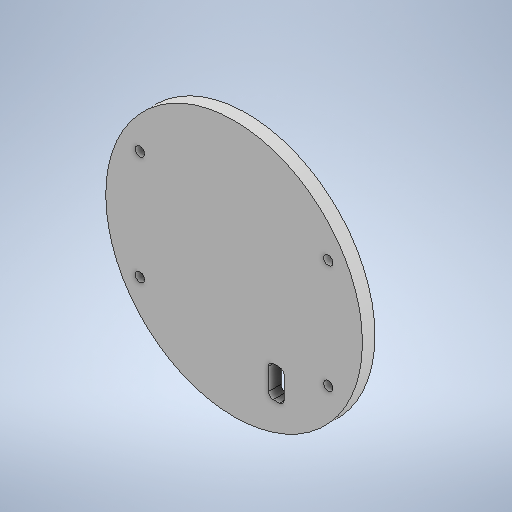
# Autodesk Inventor part: lower-plate
Saved by Autodesk Inventor 2025 (Build 290162000, 162)
## iProperties
Created: 2024-05-27
Part Number: lower-plate
Material: Generic
Document SubType Name: Modeling
Designer: hifzh
Density: 1 g/cm^3
Appearance: Default
Author: hifzh
## iProperties of the stored document lower-plate_3DPrint.ipt
Created: 2024-05-27
Part Number: lower-plate_3DPrint
Material: Generic
Document SubType Name: Modeling
Designer: hifzh
Density: 1 g/cm^3
Appearance: Default
Author: hifzh
Autodesk Inventor part; units mm, degrees
ref_plane "YZ Plane" through (0, 0, 0) normal (1, 0, 0) x (0, 1, 0)
sketch "Sketch1" plane through (0, 0, 0) normal (0, 0, 1) x (1, 0, 0)
  circle A0 centre (0, 0) radius 41
  circle A1 centre (0, 0) radius 17.705
  circle A2 centre (0, 0) radius 15
  circle A3 centre (0, 15) radius 0.75
  circle A4 centre (-10.6066, 10.6066) radius 0.75
  circle A5 centre (-15, 0) radius 0.75
  circle A6 centre (-10.6066, -10.6066) radius 0.75
  circle A7 centre (0, -15) radius 0.75
  circle A8 centre (10.6066, -10.6066) radius 0.75
  circle A9 centre (15, 0) radius 0.75
  circle A10 centre (10.6066, 10.6066) radius 0.75
  dimension "d4" = 30
  dimension "d0" = 82
  dimension "d3" = 35.41
  dimension "d5" = 1.5
  dimension "d6" = 360
  constraints: 10 centre point, 3 coincident, 1 vertical alignment, 19 other
  measures "d0" diameter of A0
  measures "d3" diameter of A1
  measures "d5" diameter of A3
sketch "Sketch2" plane through (0, 0, 0) normal (0, 0, 1) x (1, 0, 0)
  circle A0 centre (-30.094, -17.375) radius 1.5
  circle A1 centre (-30.094, 17.375) radius 1.5
  circle A2 centre (30.094, 17.375) radius 1.5
  circle A3 centre (30.094, -17.375) radius 1.5
  point P0 (0, 0)
  dimension "d7" = 3
  dimension "d8" = 3
  dimension "d9" = 3
  dimension "d10" = 3
  dimension "d11" = 17.375
  dimension "d12" = 30.094
  dimension "d13" = 30.094
  dimension "d14" = 17.375
  dimension "d15" = 17.375
  dimension "d16" = 30.094
  dimension "d17" = 17.375
  dimension "d18" = 30.094
  constraints: 4 centre point
  measures "d7" diameter of A0
  measures "d8" diameter of A1
  measures "d9" diameter of A2
  measures "d10" diameter of A3
  measures "d11" vertical distance of point (0, 0) A1.centre
  measures "d12" horizontal distance of point (0, 0) A1.centre
  measures "d13" horizontal distance of point (0, 0) A2.centre
  measures "d14" vertical distance of point (0, 0) A2.centre
  measures "d15" vertical distance of point (0, 0) A3.centre
  measures "d16" horizontal distance of point (0, 0) A3.centre
  measures "d17" vertical distance of point (0, 0) A0.centre
  measures "d18" horizontal distance of point (0, 0) A0.centre
extrude "Extrusion1" add sketch "Sketch1" against normal blind 4 contours A0 | A1 | A2 A9 | A2 A9 | A9 A2 A8 A7 A6 A5 A4 A3 A10 | A10 A2 | A2 A10 | A8 A2 | A2 A8 | A3 A2 | A2 A3 | A7 A2 | A2 A7 | A4 A2 | A2 A4 | A6 A2 | A2 A6 | A5 A2 | A2 A5
extrude "Extrusion2" cut sketch "Sketch2" against normal blind 4
ref_plane "Work Plane1" through (0, 0, -4) normal (0, 0, 1) x (1, 0, 0)
ref_plane "Work Plane2" through (0, 0, -4) normal (0, 0, 1) x (1, 0, 0)
ref_plane "Work Plane3" through (0, 0, 0) normal (0, 0, 1) x (1, 0, 0)
sketch "Sketch5" plane through (0, 0, 0) normal (0, 0, 1) x (1, 0, 0)
  line L0 (11, -30) -> (16, -30)
  line L1 (16, -30) -> (16, -20)
  line L2 (16, -20) -> (11, -20)
  line L3 (11, -20) -> (11, -30)
  point P0 (0, 0)
  point P1 (13.5, -20)
  point P2 (13.5, -30)
  point P3 (16, -25)
  dimension "d44" = 5
  dimension "d45" = 10
  dimension "d52" = 11
  dimension "d53" = 20
  constraints: 8 end point, 3 midpoint, 2 parallel, 1 horizontal, 1 perpendicular
  measures "d44" distance of L1.end L2.end
  measures "d45" distance of point (13.5, -20) point (13.5, -30)
  measures "d52" distance from line of point (0, 0) L3
  measures "d53" distance from line of point (0, 0) L2
extrude "Extrusion5" cut sketch "Sketch5" against normal blind 4
fillet "Fillet1" radius 1.5 4 edges at (11, -20, -2) (11, -30, -2) (16, -20, -2) (16, -30, -2)
ref_plane "Work Plane6" through (0, 0, -4) normal (0, 0, -1) x (-1, 0, 0)
sketch "Sketch10" plane through (0, 0, -4) normal (0, 0, -1) x (-1, 0, 0)
  circle A0 centre (0, 0) radius 1
  dimension "d71" = 2
  constraints: 1 centre point, 1 coincident
  measures "d71" diameter of A0
extrude "Extrusion10" add sketch "Sketch10" along normal blind 10
body "Solid1"
